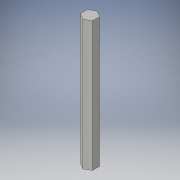
# Autodesk Inventor part: 3_8_plastic_pipe
Saved by Autodesk Inventor 2016 SP1 (Build 200210100, 210)
## iProperties
Created: 2015-11-22
Part Number: 3_8_plastic_pipe
Material: Generic
Document SubType Name: Modeling
Designer: steele
Density: 1 g/cm^3
Appearance: Default
Author: steele
Autodesk Inventor part; units mm, degrees
ref_plane "YZ Plane" through (0, 0, 0) normal (1, 0, 0) x (0, 1, 0)
ref_plane "XZ Plane" through (0, 0, 0) normal (0, 1, 0) x (-1, 0, 0)
ref_plane "XY Plane" through (0, 0, 0) normal (0, 0, 1) x (1, 0, 0)
sketch "Sketch1" plane through (0, 0, 0) normal (0, 1, 0) x (-1, 0, 0)
  line L0 (0, -5.4993) -> (-4.7625, -2.7496)
  line L1 (-4.7625, -2.7496) -> (-4.7625, 2.7496)
  line L2 (-4.7625, 2.7496) -> (0, 5.4993)
  line L3 (0, 5.4993) -> (4.7625, 2.7496)
  line L4 (4.7625, 2.7496) -> (4.7625, -2.7496)
  line L5 (4.7625, -2.7496) -> (0, -5.4993)
  point P0 (0, 0)
  point P1 (0, 0)
  dimension "d0" = 9.525
  constraints: 12 end point, 1 coincident, 13 other
  measures "d0" distance between parallel lines of L4 L1
extrude "Extrusion1" add sketch "Sketch1" along normal blind 101.6
body "Solid1"
